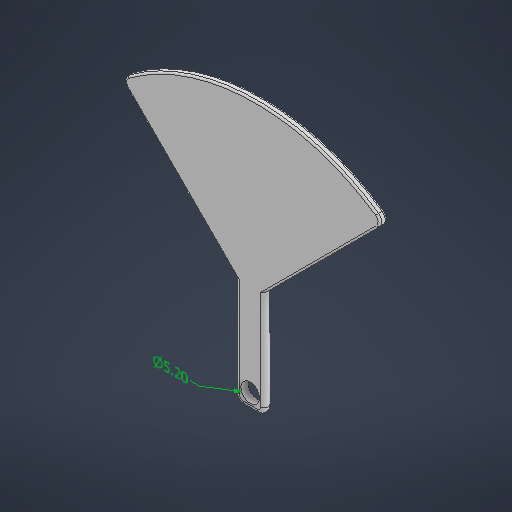
# Autodesk Inventor part: Part1#2
Saved by Autodesk Inventor 2026.2 (Build 302298010, 298A)
## iProperties
Created: 2026-04-14
Part Number: Part1#2
Material: Generic
Document SubType Name: Modeling
Designer: lenovo
Density: 1 g/cm^3
Appearance: Default
Author: lenovo
Autodesk Inventor part; units mm, degrees
ref_plane "YZ Plane" through (0, 0, 0) normal (1, 0, 0) x (0, 1, 0)
ref_plane "XZ Plane" through (0, 0, 0) normal (0, 1, 0) x (-1, 0, 0)
ref_plane "XY Plane" through (0, 0, 0) normal (0, 0, 1) x (1, 0, 0)
sketch "Sketch1" plane through (0, 0, 0) normal (0, 0, 1) x (1, 0, 0)
  line L0 (-4, 0) -> (4, 0)
  line L1 (-4, 0) -> (-4, 30)
  line L2 (4, 0) -> (4, 30)
  arc A0 (37.2135, 63.2135) -> (-35.9097, 61.9097) centre (1.5, 15) ccw
  line L3 (4, 30) -> (37.2135, 63.2135)
  line L4 (4, 30) -> (59.6428, 30) construction
  line L5 (-4, 30) -> (-35.9097, 61.9097)
  point P0 (0, 0)
  dimension "d0" = 8
  dimension "d1" = 30
  dimension "d2" = 120
  dimension "d3" = 30
  dimension "d4" = 45
  dimension "d6" = 135
  constraints: 12 end point, 2 horizontal, 2 point on circle, 2 vertical, 1 centre point, 1 midpoint
  measures "d0" distance of L0.start L0.end
  measures "d1" distance of L0.start L1.end
  measures "d2" diameter of A0
  measures "d3" distance of L0.end L2.end
  measures "d4" angle of L4 L3
  measures "d6" angle of L4 L5
extrude "Extrusion1" add sketch "Sketch1" along normal blind 2
sketch "Sketch2" plane through (0, 0, 2) normal (0, 0, 1) x (1, 0, 0)
  circle A0 centre (0, 4) radius 2.6
  line L0 (-4, 0) -> (4, 0) projected
  dimension "d23" = 5.2
  dimension "d24" = 4
  constraints: 1 centre point
  measures "d23" diameter of A0
  measures "d24" distance from line of L0 A0.centre
fillet "Fillet3" radius 2 2 edges at (37.2135, 63.2135, 1) (-35.9097, 61.9097, 1)
fillet "Fillet4" radius 2 2 edges at (4, 0, 1) (-4, 0, 1)
fillet "Fillet5" radius 0.5 10 edges at (-34.8764, 61.8612, 2) (-19.1482, 45.1482, 2) (36.1167, 63.1416, 2) (19.7698, 45.7698, 2) (0.3868, 74.9897, 2) (-34.8764, 61.8612, 0) (-19.1482, 45.1482, 0) (36.1167, 63.1416, 0) (19.7698, 45.7698, 0) (0.3868, 74.9897, 0)
extrude "Extrusion5" cut sketch "Sketch2" against normal blind 2
fillet "Fillet6" radius 1 10 edges at (3.4142, 0.5858, 2) (0, 0, 2) (-3.4142, 0.5858, 2) (-4, 16.3536, 2) (4, 16.3536, 2) (3.4142, 0.5858, 0) (0, 0, 0) (-3.4142, 0.5858, 0) (-4, 16.3536, 0) (4, 16.3536, 0)
equation "\"d3\" = d1"
body "Solid1"
